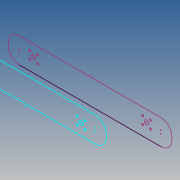
# Autodesk Inventor part: боковая стенка
Saved by Autodesk Inventor 2020 (Build 240168000, 168)
## iProperties
Created: 2021-06-26
Part Number: боковая стенка
Material: Типовые
Document SubType Name: Modeling
Designer: Петров Иван
Density: 1 g/cm^3
Appearance: По умолчанию
Mass: 28.522 g
Surface Area: 210.36 cm^2
Volume: 28.522 cm^3
Author: Петров Иван
Autodesk Inventor part; units mm, degrees
ref_plane "YZ Plane" through (0, 0, 0) normal (1, 0, 0) x (0, 1, 0)
ref_plane "XZ Plane" through (0, 0, 0) normal (0, 1, 0) x (-1, 0, 0)
ref_plane "XY Plane" through (0, 0, 0) normal (0, 0, 1) x (1, 0, 0)
sketch "Эскиз4" plane through (0, 0, 0) normal (0, 0, 1) x (1, 0, 0)
  arc A0 (-128.0581, -24.7499) -> (-111.2416, -42.0003) centre (-110.8018, -24.7496) ccw
  arc A1 (-111.2419, -3) -> (-128.0581, -20.2507) centre (-110.8018, -20.2507) ccw
  line L0 (-128.0581, -22.5003) -> (-128.0581, -24.6843)
  line L1 (-128.0581, -20.3163) -> (-128.0581, -22.5003)
  arc A2 (108.7577, -42.0003) -> (125.5742, -24.7499) centre (108.3179, -24.7496) ccw
  line L2 (125.5743, -24.6843) -> (125.5743, -20.2507)
  arc A3 (125.5743, -20.2507) -> (108.758, -3) centre (108.318, -20.2507) ccw
  line L3 (-111.2419, -3) -> (108.7581, -3)
  line L4 (-111.2416, -42.0003) -> (108.7577, -42.0003)
  circle A4 centre (-88.7419, -20.5) radius 3.4
  circle A5 centre (-94.7523, -26.5104) radius 1.5
  circle A6 centre (-82.7315, -14.4896) radius 1.5
  circle A7 centre (-94.7523, -14.4896) radius 1.5
  circle A8 centre (-82.7315, -26.5104) radius 1.5
  circle A9 centre (86.2581, -20.5) radius 3.4
  circle A10 centre (80.2477, -26.5104) radius 1.5
  circle A11 centre (92.2685, -26.5104) radius 1.5
  circle A12 centre (92.2685, -14.4896) radius 1.5
  circle A13 centre (80.2477, -14.4896) radius 1.5
  line L5 (-128.0581, -24.6843) -> (-128.0581, -24.7499)
  line L6 (-128.0581, -20.2507) -> (-128.0581, -20.3163)
  line L7 (125.5743, -24.6843) -> (125.5742, -24.7499)
  point P0 (0, 0)
  constraints: 16 end point, 14 centre point, 8 point on circle, 1 point on line
extrude "Выдавливание4" add sketch "Эскиз4" along normal blind 3
